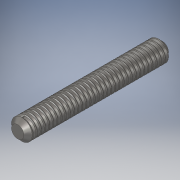
# Autodesk Inventor part: Thread
Saved by Autodesk Inventor 2017 (Build 210142000, 142)
## iProperties
Created: 2016-06-17
Part Number: Thread
Material: Steel, Carbon
Document SubType Name: Modeling
Designer: Dakota Marin
Density: 7.85 g/cm^3
Appearance: Semi-Polished
Author: Dakota Marin
Autodesk Inventor part; units mm, degrees
ref_plane "YZ Plane" through (0, 0, 0) normal (1, 0, 0) x (0, 1, 0)
ref_plane "XZ Plane" through (0, 0, 0) normal (0, 1, 0) x (-1, 0, 0)
ref_plane "XY Plane" through (0, 0, 0) normal (0, 0, 1) x (1, 0, 0)
sketch "Sketch1" plane through (0, 0, 0) normal (0, 0, 1) x (1, 0, 0)
  circle A0 centre (0, 0) radius 7.5
  dimension "d0" = 15
  constraints: 1 centre point, 1 coincident
  measures "d0" diameter of A0
extrude "Extrusion1" add sketch "Sketch1" along normal blind 105
chamfer "Chamfer1" distance 3 angle 45 2 edges at (-7.5, 0, 105) (-7.5, 0, 0)
sketch "Sketch2" plane through (0, 0, 0) normal (1, 0, 0) x (0, 1, 0)
  line L0 (-7.5, 0) -> (7.5, 0) projected
  line L1 (7.5, 0) -> (7.5, -2)
  line L2 (7.5, -2) -> (6.5, -1)
  line L3 (7.5, 0) -> (6.5, -1)
  point P0 (0, 0)
  dimension "d5" = 45
  dimension "d6" = 45
  dimension "d7" = 2
  constraints: 6 end point, 1 vertical
  measures "d5" angle of L1 L2
  measures "d6" angle of L1 L3
  measures "d7" distance of L0.end L1.end
coil "Coil1" sketch "Sketch2" operation cut axis through (0, 0, -10) along (0, 0, 1) pitch 3 turns 34 hand right
body "Solid1"
